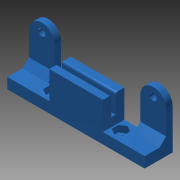
# Autodesk Inventor part: GT2 grip v2
Saved by Autodesk Inventor 2013 SP2 (Build 170200200, 200)
## iProperties
Created: 2017-01-29
Part Number: GT2 grip v2
Material: Generic
Document SubType Name: Modeling
Designer: Herman de Vries
Density: 1 g/cm^3
Mass: 8.9464 g
Surface Area: 55.9898 cm^2
Volume: 8.9464 cm^3
Author: Herman de Vries
Autodesk Inventor part; units mm, degrees
ref_plane "YZ Plane" through (0, 0, 0) normal (1, 0, 0) x (0, 1, 0)
ref_plane "XZ Plane" through (0, 0, 0) normal (0, 1, 0) x (-1, 0, 0)
ref_plane "XY Plane" through (0, 0, 0) normal (0, 0, 1) x (1, 0, 0)
sketch "Sketch1" plane through (0, 0, 0) normal (0, 0, 1) x (1, 0, 0)
  line L0 (0, 0) -> (40, 0)
  line L1 (40, 0) -> (40, 10)
  line L2 (40, 10) -> (0, 10)
  line L3 (0, 10) -> (0, 0)
  circle A0 centre (4, 5) radius 1.6
  circle A1 centre (36, 5) radius 1.6
  line L4 (0, 0) -> (-12, 0)
  line L5 (-12, 0) -> (-12, 13)
  line L6 (-12, 13) -> (0, 13)
  line L7 (0, 13) -> (0, 0)
  line L8 (40, 0) -> (52, 0)
  line L9 (52, 0) -> (52, 13)
  line L10 (52, 13) -> (40, 13)
  line L11 (40, 13) -> (40, 0)
  point P0 (0, 5)
  dimension "d0" = 40
  dimension "d1" = 10
  dimension "d22" = 3.2
  dimension "d23" = 3.2
  dimension "d24" = 4
  dimension "d25" = 4
  dimension "d43" = 12
  dimension "d44" = 12
  dimension "d45" = 13
  dimension "d46" = 13
  constraints: 24 end point, 6 parallel, 3 horizontal, 3 perpendicular, 2 centre point, 2 horizontal alignment, 1 midpoint
  measures "d0" distance of L2.end L1.end
  measures "d1" distance of L1.end L0.end
  measures "d22" diameter of A0
  measures "d23" diameter of A1
  measures "d24" distance from line of L3 A0.centre
  measures "d25" distance from line of L1 A1.centre
  measures "d43" distance of L5.end L6.end
  measures "d44" distance of L10.end L9.end
  measures "d45" distance of L9.end L8.end
  measures "d46" distance of L4.end L5.end
extrude "Extrusion1" add sketch "Sketch1" along normal blind 5 contours L3 L2 L1 L0
extrude "Extrusion5" add sketch "Sketch1" along normal blind 5 contours L4 L5 L6 L7 L3 | L1 L11 L10 L9 L8
sketch "Sketch2" plane through (0, 0, 5) normal (0, 0, 1) x (1, 0, 0)
  line L0 (40, 10) -> (0, 10) projected
  line L1 (0, 0) -> (40, 0) projected
  line L2 (7.5, 10) -> (32.5, 10)
  line L3 (32.5, 10) -> (32.5, 6)
  line L4 (32.5, 6) -> (7.5, 6)
  line L5 (7.5, 6) -> (7.5, 10)
  line L6 (7.5, 0) -> (32.5, 0)
  line L7 (32.5, 0) -> (32.5, 4)
  line L8 (32.5, 4) -> (7.5, 4)
  line L9 (7.5, 4) -> (7.5, 0)
  line L10 (0, 13) -> (-12, 13) projected
  line L11 (52, 13) -> (40, 13) projected
  line L12 (-12, 13) -> (0, 13)
  line L13 (0, 13) -> (0, 10)
  line L14 (0, 10) -> (-12, 10)
  line L15 (-12, 10) -> (-12, 13)
  line L16 (52, 13) -> (40, 13)
  line L17 (40, 13) -> (40, 10)
  line L18 (40, 10) -> (52, 10)
  line L19 (52, 10) -> (52, 13)
  point P0 (20, 10)
  point P1 (20, 10)
  point P2 (20, 0)
  point P3 (20, 0)
  dimension "d14" = 25
  dimension "d15" = 25
  dimension "d31" = 2
  dimension "d32" = 4
  dimension "d33" = 4
  constraints: 32 end point, 8 parallel, 4 horizontal, 4 midpoint, 4 perpendicular, 2 coincident, 2 point on line
  measures "d14" distance of L2.start L2.end
  measures "d15" distance between parallel lines of L9 L7
  measures "d31" distance between parallel lines of L8 L4
  measures "d32" distance of L2.end L3.end
  measures "d33" distance of L6.end L7.end
extrude "Extrusion2" add sketch "Sketch2" along normal blind 13 contours L3 L4 L5 L0 | L9 L8 L7 L1
fillet "Fillet1" radius 1 2 edges at (20, 6, 18) (20, 4, 18)
sketch "Sketch3" plane through (0, 0, 5) normal (0, 0, 1) x (1, 0, 0)
  circle A0 centre (4, 5) radius 1.6 projected
  circle A1 centre (36, 5) radius 1.6 projected
  line L0 (6.75, 6.5877) -> (6.75, 3.4123)
  line L1 (6.75, 3.4123) -> (4, 1.8246)
  line L2 (4, 1.8246) -> (1.25, 3.4123)
  line L3 (1.25, 3.4123) -> (1.25, 6.5877)
  line L4 (1.25, 6.5877) -> (4, 8.1754)
  line L5 (4, 8.1754) -> (6.75, 6.5877)
  line L6 (33.25, 6.5877) -> (36, 8.1754)
  line L7 (36, 8.1754) -> (38.75, 6.5877)
  line L8 (38.75, 6.5877) -> (38.75, 3.4123)
  line L9 (38.75, 3.4123) -> (36, 1.8246)
  line L10 (36, 1.8246) -> (33.25, 3.4123)
  line L11 (33.25, 3.4123) -> (33.25, 6.5877)
  point P0 (0, 0)
  dimension "d39" = 5.5
  dimension "d40" = 5.5
  constraints: 24 end point, 2 coincident, 2 vertical, 26 other
  measures "d39" distance between parallel lines of L0 L3
  measures "d40" distance between parallel lines of L8 L11
extrude "Extrusion3" cut sketch "Sketch3" against normal blind 3
sketch "Sketch4" plane through (0, 0, 5) normal (0, 0, 1) x (1, 0, 0)
  line L0 (7.5, 6) -> (7.5, 10) projected
  line L1 (32.5, 4) -> (32.5, 0) projected
  line L2 (7.5, 6) -> (32.5, 6)
  line L3 (32.5, 6) -> (32.5, 4)
  line L4 (32.5, 4) -> (7.5, 4)
  line L5 (7.5, 4) -> (7.5, 6)
  point P0 (0, 0)
  constraints: 8 end point, 2 parallel, 1 horizontal, 1 perpendicular
extrude "Extrusion4" add sketch "Sketch4" along normal blind 4
extrude "Extrusion7" add sketch "Sketch2" along normal blind 20 contours L13 L14 L15 L10 | L19 L18 L17 L11
sketch "Sketch5" plane through (-12, 10, 5) normal (0, -1, 0) x (1, 0, 0)
  circle A0 centre (6, 16) radius 1.6
  circle A1 centre (58, 16) radius 1.6
  line L0 (0, 20) -> (12, 20) projected
  line L1 (52, 20) -> (64, 20) projected
  point P0 (15, -5)
  point P1 (6, 20)
  point P2 (58, 20)
  dimension "d49" = 3.2
  dimension "d50" = 3.2
  dimension "d56" = 4
  constraints: 2 centre point, 2 midpoint, 2 vertical alignment, 1 horizontal alignment
  measures "d49" diameter of A0
  measures "d50" diameter of A1
  measures "d56" distance from line of A0.centre L0
extrude "Extrusion6" cut sketch "Sketch5" against normal blind 5
chamfer "Chamfer2" distance 3 angle 45 2 edges at (-6, 10, 5) (46, 10, 5)
fillet "Fillet2" radius 6 4 edges at (0, 11.5, 25) (-12, 11.5, 25) (40, 11.5, 25) (52, 11.5, 25)
equation "\"d23\" = d22"
equation "\"d44\" = d43"
equation "\"d45\" = d46"
equation "\"d15\" = d14"
equation "\"d32\" = d33"
equation "\"d40\" = d39"
equation "\"d50\" = d49"
body "Solid1"
